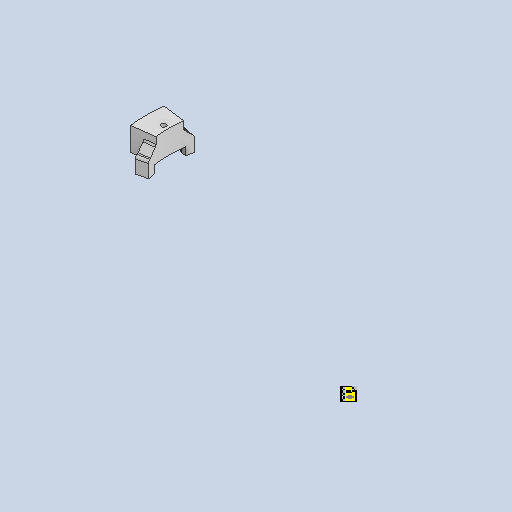
# Autodesk Inventor part: Spacer (make 5)
Saved by Autodesk Inventor 2025.1 (Build 291241020, 241B)
## iProperties
Created: 2024-12-11
Part Number: Spacer (make 5)
Material: Generic
Document SubType Name: Modeling
Designer: jdl5984
Density: 1 g/cm^3
Appearance: Default
Author: jdl5984
Autodesk Inventor part; units mm, degrees
ref_plane "YZ Plane" through (0, 0, 0) normal (1, 0, 0) x (0, 1, 0)
ref_plane "XZ Plane" through (0, 0, 0) normal (0, 1, 0) x (-1, 0, 0)
ref_plane "XY Plane" through (0, 0, 0) normal (0, 0, 1) x (1, 0, 0)
sketch "Sketch1" plane through (0, 0, 0) normal (0, 1, 0) x (-1, 0, 0)
  circle A0 centre (0, 0) radius 2.6543
  circle A1 centre (0, 0) radius 12.7 construction
  circle A2 centre (-120.65, 0) radius 120.65 construction
  arc A3 (5.2635, 16.5768) -> (5.2635, -16.5768) centre (-120.65, 0) ccw
  circle A4 centre (-120.65, 0) radius 92.075 construction
  line L0 (-120.65, 0) -> (17.8548, -18.2345)
  line L1 (-120.65, 0) -> (17.8548, 18.2345)
  line L2 (95.25, 0) -> (-260.35, 0) construction
  arc A5 (-6.5724, -15.0186) -> (-6.5724, 15.0186) centre (-120.65, 0) ccw
  circle A6 centre (-120.65, 0) radius 139.7
  line L3 (166.37, 0) -> (-331.47, 0) projected
  circle A7 centre (-120.65, 0) radius 115.062
  line L4 (-120.65, 0) -> (15.7386, 30.2366)
  line L5 (-120.65, 0) -> (15.7386, -30.2366)
  line L6 (-120.65, 0) -> (4.955, 18.7718)
  line L7 (-120.65, 0) -> (4.955, -18.7718)
  point P0 (-5.588, 0)
  point P1 (-8.3154, -24.904)
  point P2 (3.3396, -27.4878)
  point P3 (3.3396, 27.4878)
  point P4 (-8.3154, 24.904)
  point P5 (-6.5724, 15.0186)
  point P6 (-6.8519, 17.0072)
  point P7 (-6.8519, -17.0072)
  dimension "d4" = 241.3
  dimension "d0" = 5.3086
  dimension "d1" = 25.4
  dimension "d5" = 254
  dimension "d6" = 184.15
  dimension "d7" = 7.5
  dimension "d8" = 7.5
  dimension "d9" = 5.588
  dimension "d10" = 279.4
  dimension "d11" = 115.062
  dimension "d12" = 355.6
  dimension "d13" = 25
  dimension "d14" = 12.5
  dimension "d22" = 17
  dimension "d23" = 8.5
  constraints: 14 end point, 12 point on circle, 7 coincident, 6 centre point, 4 point on line, 1 collinear, 1 horizontal, 1 horizontal alignment, 5 other
  measures "d0" diameter of A0
  measures "d1" diameter of A1
  measures "d5" diameter of A3
  measures "d6" diameter of A4
  measures "d7" angle of L0 L2
  measures "d8" angle of L1 L2
  measures "d9" distance of point (-5.588, 0) point (0, 0)
  measures "d10" diameter of A6
  measures "d11" radius of A5
  measures "d12" distance of L2.start L2.end
  measures "d13" angle of L4 L5
  measures "d14" angle of L4 L2
  measures "d22" angle of L6 L7
  measures "d23" angle of L3 L7
extrude "Extrusion1" add sketch "Sketch1" along normal blind 25.4 contours L3 A6 L0 A5 A0 | A0 L3 A5 L1 A6
extrude "Extrusion2" add sketch "Sketch1" along normal mid plane 17.018 contours L7 A3 L5 A7 | A7 L4 A3 L6
extrude "Extrusion3" add sketch "Sketch1" along normal blind 8.509 contours L0 A3 L7 A7 | A7 L6 A3 L1
chamfer "Chamfer1" distance 8.382 angle 45 2 edges at (0.6544, 8.509, 15.7977) (0.6544, 8.509, -15.7977)
fillet "Fillet1" radius 3.175 6 edges at (2.4879, 8.509, 26.1959) (2.0373, 8.509, -24.07) (2.0373, 8.509, 24.07) (0.6544, 16.891, 15.7977) (0.6544, 16.891, -15.7977) (2.4879, 8.509, -26.1959)
fillet "Fillet2" radius 6.35 2 edges at (-4.955, -4.2545, 18.7718) (-4.955, -4.2545, -18.7718)
equation "\"d14\" = 0.5 * d13"
equation "\"d23\" = 0.5 * d22"
body "Solid1"
